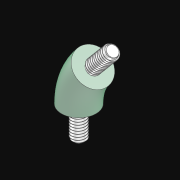
# Autodesk Inventor part: Rubber Link bent
Saved by Autodesk Inventor 2021.2 (Build 252289000, 289)
## iProperties
Created: 2021-02-24
Part Number: Rubber Link bent
Material: Generic
Document SubType Name: Modeling
Designer: yuany
Density: 1 g/cm^3
Appearance: Default
Author: yuany
Autodesk Inventor part; units mm, degrees
ref_plane "YZ Plane" through (0, 0, 0) normal (1, 0, 0) x (0, 1, 0)
ref_plane "XZ Plane" through (0, 0, 0) normal (0, 1, 0) x (-1, 0, 0)
ref_plane "XY Plane" through (0, 0, 0) normal (0, 0, 1) x (1, 0, 0)
sketch "Sketch1" plane through (0, 0, 0) normal (0, 1, 0) x (-1, 0, 0)
  circle A0 centre (0, 0) radius 5.207
  dimension "d0" = 10.414
  constraints: 1 centre point, 1 coincident
  measures "d0" diameter of A0
sketch "Sketch2" plane through (0, 0, 0) normal (0, 0, 1) x (1, 0, 0)
  arc A0 (4.256, 11.6932) -> (0, 0) centre (18.1914, 0) ccw
  line L0 (0, 0) -> (6.35, 0) construction
  line L1 (4.256, 11.6932) -> (9.1204, 7.6115) construction
  dimension "BendAngle" = 40
  dimension "d2" = 12.7
  dimension "d3" = 6.35
  constraints: 4 end point, 2 line through centre, 2 point on circle, 1 centre point, 1 equal length, 1 horizontal
  measures "BendAngle" angle of L0 L1
  measures "d3" distance of L1.start L1.end
sweep "Rubber" add profiles "Sketch1" path "Sketch2"
sketch "Sketch3" plane through (4.256, 11.6932, 0) normal (0.6427876, 0.7660444, 0) x (0, 0, -1)
  circle A0 centre (0, 0) radius 1.5621
  point P0 (0, -4.256)
  dimension "d6" = 3.1242
  constraints: 1 centre point
  measures "d6" diameter of A0
extrude "Extrusion1" add sketch "Sketch3" along normal blind 9.271
sketch "Sketch4" plane through (0, 0, 0) normal (0, -1, 0) x (1, 0, 0)
  circle A0 centre (0, 0) radius 1.5621
  dimension "d9" = 3.1242
  constraints: 1 centre point, 1 coincident
  measures "d9" diameter of A0
extrude "Extrusion2" add sketch "Sketch4" along normal blind 9.271
sketch "Sketch5" plane through (0, 0, 0) normal (0, 0, 1) x (1, 0, 0)
  line L0 (1.5621, 0) -> (1.5621, -9.271) projected
  line L1 (1.5621, -9.1948) -> (1.5621, -9.9123)
  line L2 (1.5621, -9.9123) -> (2.0955, -9.6044)
  line L3 (2.0955, -9.6044) -> (2.0955, -9.5028)
  line L4 (2.0955, -9.5028) -> (1.5621, -9.1948)
  line L5 (-1.5621, -9.271) -> (1.5621, -9.271) projected
  point P0 (0, 0)
  dimension "d12" = 0.1016
  dimension "d13" = 60
  dimension "d14" = 0.5334
  dimension "d15" = 0.0762
  constraints: 8 end point, 1 collinear, 1 equal length, 1 parallel, 1 point on line
  measures "d12" distance of L2.end L3.end
  measures "d13" angle of L4 L2
  measures "d14" distance between parallel lines of L3 L1
  measures "d15" distance from line of L1.start L5
coil "Coil1" sketch "Sketch5" operation add axis through (0, -10, 0) along (0, 1, 0) pitch 0.7874 turns 13.387097 hand right
sketch "Sketch6" plane through (0, 0, 0) normal (0, 0, 1) x (1, 0, 0)
  line L0 (11.3629, 17.7327) -> (11.8241, 18.2824)
  line L1 (11.8241, 18.2824) -> (12.0348, 17.7036)
  line L2 (12.0348, 17.7036) -> (11.9695, 17.6258)
  line L3 (11.9695, 17.6258) -> (11.3629, 17.7327)
  line L4 (11.4119, 17.7911) -> (9.0186, 19.7993) projected
  point P0 (0, 0)
  dimension "d24" = 0.1016
  dimension "d25" = 0.5334
  dimension "d26" = 60
  dimension "d27" = 0.0762
  constraints: 9 end point, 1 equal length, 1 parallel, 1 perpendicular, 1 point on line
  measures "d24" distance of L1.end L2.end
  measures "d25" distance between parallel lines of L0 L2
  measures "d26" angle of L3 L1
  measures "d27" distance from line of L4 L0.start
coil "Coil2" sketch "Sketch6" operation add axis through (10.2153, 18.7952, 0) along (-0.6427876, -0.7660444, 0) pitch 0.7874 turns 13.387097 hand right
sketch "Sketch7" plane through (0, 0, 0) normal (0, 0, 1) x (1, 0, 0)
  line L0 (2.573, -8.1966) -> (3.9042, -10.6838)
  line L1 (3.9042, -10.6838) -> (1.4986, -10.2553)
  line L2 (0, 0) -> (0, -13.1029)
  line L3 (1.4986, -10.2553) -> (1.4986, -9.271)
  line L4 (1.5621, -9.271) -> (1.5621, -9.9123) projected
  line L5 (1.4986, -9.271) -> (2.573, -8.1966)
  line L6 (0.6156, -9.271) -> (1.5621, -9.271) projected
  dimension "d37" = 1.4986
  dimension "d38" = 135
  constraints: 10 end point, 1 point on line, 1 vertical
  measures "d37" distance between parallel lines of L2 L3
  measures "d38" angle of L5 L3
revolve "Revolution1" cut sketch "Sketch7" angle 360 about axis through (0, 0, 0) along (0, -1, 0)
sketch "Sketch8" plane through (0, 0, 0) normal (0, 0, 1) x (1, 0, 0)
  line L0 (12.6976, 19.4221) -> (11.3633, 17.8319)
  line L1 (11.3633, 17.8319) -> (11.5049, 16.2126)
  line L2 (11.5049, 16.2126) -> (14.2785, 18.1114)
  line L3 (14.2785, 18.1114) -> (12.6976, 19.4221)
  line L4 (-9.01, -4.1166) -> (16.1784, 25.9018) projected
  line L5 (11.4119, 17.7911) -> (10.6869, 18.3995) projected
  point P0 (0, 0)
  dimension "d40" = 1.4986
  dimension "d41" = 135
  constraints: 8 end point, 1 parallel, 1 point on line
  measures "d40" distance between parallel lines of L4 L0
  measures "d41" angle of L0 L1
revolve "Revolution2" cut sketch "Sketch8" angle 360 about axis through (10.2153, 18.7952, 0) along (0.6427876, 0.7660444, 0)
body "Solid1"
